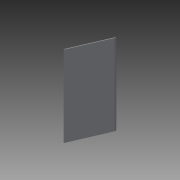
# Autodesk Inventor part: Left Abdomen
Saved by Autodesk Inventor 2014 (Build 180170000, 170)
## iProperties
Created: 2015-08-01
Part Number: Left Abdomen
Material: Generic
Document SubType Name: Modeling
Designer: Devon
Density: 1 g/cm^3
Appearance: Default
Author: Devon
Autodesk Inventor part; units mm, degrees
ref_plane "YZ Plane" through (0, 0, 0) normal (1, 0, 0) x (0, 1, 0)
ref_plane "XZ Plane" through (0, 0, 0) normal (0, 1, 0) x (-1, 0, 0)
ref_plane "XY Plane" through (0, 0, 0) normal (0, 0, 1) x (1, 0, 0)
sketch "Sketch1" plane through (0, 0, 0) normal (0, 0, 1) x (1, 0, 0)
  line L0 (-24.3533, 25.6313) -> (-24.3533, -114.0687)
  line L1 (-24.3533, -114.0687) -> (64.0742, -52.1511)
  line L2 (-24.3533, -114.0687) -> (83.5967, -114.0687) construction
  line L3 (64.0742, -52.1511) -> (64.0742, 87.5489)
  line L4 (64.0742, 87.5489) -> (-24.3533, 25.6313)
  point P0 (0, 0)
  dimension "d0" = 139.7
  dimension "d1" = 107.95
  dimension "d2" = 35
  dimension "d3" = 139.7
  constraints: 10 end point, 1 equal length, 1 horizontal, 1 perpendicular, 1 vertical
  measures "d0" distance of L0.start L0.end
  measures "d1" distance of L0.end L1.end
  measures "d2" angle of L2 L1
  measures "d3" distance of L1.end L3.end
extrude "Extrusion1" add sketch "Sketch1" along normal blind 3.175
body "Solid1"
